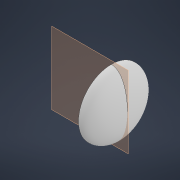
# Autodesk Inventor part: test spin toy
Saved by Autodesk Inventor 2022 (Build 260153000, 153)
## iProperties
Created: 2021-05-31
Part Number: test spin toy
Material: Generic
Document SubType Name: Modeling
Designer: sidsa
Density: 1 g/cm^3
Appearance: Default
Author: sidsa
## iProperties of the stored document test spin toy_3DPrint.ipt
Created: 2021-05-31
Part Number: test spin toy_3DPrint
Material: Generic
Document SubType Name: Modeling
Designer: sidsa
Density: 1 g/cm^3
Appearance: Default
Author: sidsa
Autodesk Inventor part; units mm, degrees
ref_plane "YZ Plane" through (0, 0, 0) normal (1, 0, 0) x (0, 1, 0)
ref_plane "XZ Plane" through (0, 0, 0) normal (0, 1, 0) x (-1, 0, 0)
sketch "Sketch1" plane through (0, 0, 0) normal (0, 0, 1) x (1, 0, 0)
  spline S0 degree 5 poles (0, 0) (1.6794, 2.0153) (3.359, 4.0308) (5.045, 6.0401) (8.3598, 9.9376) (11.7583, 13.7609) (13.4423, 15.5999) (16.701, 19.0191) (20.1453, 22.2559) (21.8214, 23.7259) (25.0365, 26.3061) (28.5489, 28.4419) (30.236, 29.2993) (33.7337, 30.596) (37.5009, 30.6259) (39.328, 30.1757) (46.3458, 26.1718) (48.9096, 17.582) (50.1746, 12.3101) (50.8057, 5.9191) (50.8, 0) knots 0 0 0 0 0 0 0.153806 0.153806 0.153806 0.29993 0.29993 0.29993 0.430709 0.430709 0.430709 0.540808 0.540808 0.540808 0.647062 0.647062 0.647062 1 1 1 1 1 1
  line L0 (0, 0) -> (50.8, 0)
  constraints: 2 end point, 1 horizontal, 1 horizontal alignment, 2 other
revolve "Revolution1" add sketch "Sketch1" angle 360 about axis through (0, 0, 0) along (1, 0, 0)
sketch "Sketch2" plane through (0, 0, 0) normal (0, 0, 1) x (1, 0, 0)
  spline S0 degree 3 poles (50.8, 0) (50.7915, 1.2047) (50.7831, 1.6058) (50.7746, 1.9265) (50.7732, 1.9785) (50.7719, 2.0283) (50.7705, 2.0765) (50.7544, 2.6401) (50.7384, 3.0178) (50.7224, 3.364) (50.7011, 3.8217) (50.6799, 4.1928) (50.6587, 4.5305) (50.6201, 5.1455) (50.5815, 5.643) (50.5428, 6.0949) (50.4656, 6.9988) (50.3883, 7.7117) (50.3111, 8.3559) (50.1566, 9.6441) (50.0021, 10.638) (49.8476, 11.5285) (49.5386, 13.3095) (49.2296, 14.6441) (48.9206, 15.8202) (48.3915, 17.8339) (47.8624, 19.3352) (47.3334, 20.6228) (46.4825, 22.6935) (45.6317, 24.1742) (44.7809, 25.3724) (43.4754, 27.211) (42.1698, 28.3556) (40.8643, 29.1314) (38.9438, 30.2726) (37.0233, 30.5927) (35.1028, 30.4491) (32.3823, 30.2457) (29.6618, 29.0931) (26.9413, 27.4085) (23.1978, 25.0904) (19.4544, 21.7489) (15.711, 17.9289) (10.474, 12.5847) (5.237, 6.2844) (0, 0) knots -2 -2 -2 -2 -1.999 -1.999 -1.999 -1.998838 -1.998838 -1.998838 -1.996943 -1.996943 -1.996943 -1.994438 -1.994438 -1.994438 -1.989876 -1.989876 -1.989876 -1.980752 -1.980752 -1.980752 -1.962504 -1.962504 -1.962504 -1.926008 -1.926008 -1.926008 -1.863518 -1.863518 -1.863518 -1.763026 -1.763026 -1.763026 -1.608832 -1.608832 -1.608832 -1.381998 -1.381998 -1.381998 -1.060681 -1.060681 -1.060681 -0.618542 -0.618542 -0.618542 0 0 0 0
  line L0 (35.9272, 30.4812) -> (35.9272, -30.5651)
  line L1 (35.9272, -30.5651) -> (67.3017, -30.5651)
  line L2 (67.3017, -30.5651) -> (67.3017, 30.4812)
  line L3 (67.3017, 30.4812) -> (35.9272, 30.4812)
  line L4 (35.9272, 30.4812) -> (-48.0614, 30.4812)
  line L5 (-48.0614, 30.4812) -> (-48.0614, -59.2628)
  line L6 (-48.0614, -59.2628) -> (35.9272, -59.2628)
  line L7 (35.9272, -59.2628) -> (35.9272, 30.4812)
  point P0 (35.9272, -30.5651)
  constraints: 16 end point, 4 perpendicular, 2 parallel, 1 horizontal, 1 vertical, 3 other
extrude "Extrusion1" cut sketch "Sketch2" along normal mid plane 127 contours L0 L7 L6 L5 L4
equation "curve S0 of \"Sketch1\": x = t; y = 0.6 ul*t*sqrt(4 ul-t*t); t from d0 to d1"
body "Solid1"
